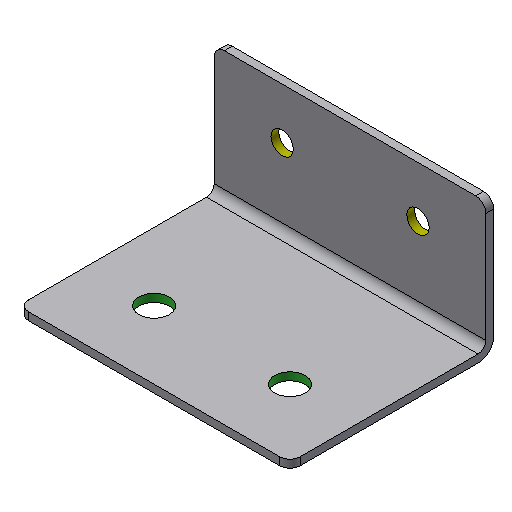
# Autodesk Inventor part: TL20240701-10130CV-002
Saved by Autodesk Inventor 2022.5 (Build 265521000, 521)
## iProperties
Category: JOINT LEG ASSY
Company: 현대 트랜시스(대유)
Created: 2023-04-20
Part Number: TL20240701-10130CV-002
Checked By: 김형민
Engr Approved By: 김시현
User Status: 2 x37
Material: SS400
Description: 0
Document SubType Name: Modeling
Mfg Approved By: 호상태
Designer: 김건휴
Stock Number: 002
Density: 7.85 g/cm^3
Appearance: Painting-RAL7035
Project: SW PJT
DETAIL: Coveryor Assembly
M/C TITLE: CJ 제일제당 협동로봇 포장시스탬 PILOT 장비
PARTS NAME: Bracket
SPECIFICATION: TA20221101-CV200000-015
DocNumber: 221118_Standard_v1
Folder: .\
VDS_Category: 엔지니어링
Detail Description: Processed products
Title: BRACKET
Subject: SW차종 시트조립라인
Author: 김건휴
Revision Number: A
Autodesk Inventor part; units mm, degrees
ref_plane "YZ Plane" through (0, 0, 0) normal (1, 0, 0) x (0, 1, 0)
ref_plane "XZ Plane" through (0, 0, 0) normal (0, 1, 0) x (-1, 0, 0)
ref_plane "XY Plane" through (0, 0, 0) normal (0, 0, 1) x (1, 0, 0)
sketch "스케치9" plane through (0, 0, 0) normal (1, 0, 0) x (0, 1, 0)
  line L0 (2.3, 0) -> (0, 0)
  line L1 (0, 0) -> (0, 60)
  line L2 (0, 60) -> (2.3, 60)
  line L3 (2.3, 60) -> (2.3, 0)
  line L4 (0, 0) -> (40, 0)
  line L5 (40, 0) -> (40, 2.3)
  line L6 (40, 2.3) -> (0, 2.3)
  line L7 (0, 2.3) -> (0, 0)
  point P0 (2.3, 2.3)
  dimension "d40" = 2.3
  dimension "d41" = 2.3
  dimension "d42" = 60
  dimension "d43" = 40
  constraints: 16 end point, 4 parallel, 2 horizontal, 2 perpendicular, 1 coincident
  measures "d40" distance of L4.end L5.end
  measures "d41" distance of L1.end L2.end
  measures "d42" distance of point (0, 0) L1.end
  measures "d43" distance of L0.end L4.end
extrude "돌출4" add sketch "스케치9" along normal blind 80
sketch "스케치10" plane through (0, 2.3, 2.3) normal (0, 0, 1) x (1, 0, 0)
  line L0 (0, 37.7) -> (0, 0) projected
  line L1 (80, 37.7) -> (80, 0) projected
  line L2 (0, -2.3) -> (80, -2.3) projected
  point P0 (20, 22.7)
  point P1 (60, 22.7)
  dimension "d46" = 20
  dimension "d47" = 20
  dimension "d48" = 25
  constraints: 1 horizontal alignment
  measures "d46" distance from line of point (20, 22.7) L0
  measures "d47" distance from line of L1 point (60, 22.7)
  measures "d48" distance from line of point (20, 22.7) L2
hole "구멍3" at (20, 25, 2.3) at (60, 25, 2.3) direction (0, 0, -1) diameter 6.6 end through all clearance for "Slotted Cheese Head Screw ISO 1207" size "M6" standard "ISO"
sketch "스케치11" plane through (0, 2.3, 60) normal (0, 1, 0) x (1, 0, 0)
  line L0 (0, 57.7) -> (0, 0) projected
  line L1 (0, 0) -> (80, 0) projected
  point P0 (0, 60)
  point P1 (20, 20)
  point P2 (60, 20)
  dimension "d56" = 20
  dimension "d57" = 40
  dimension "d58" = 20
  constraints: 1 horizontal alignment
  measures "d56" distance from line of point (20, 20) L0
  measures "d57" distance of point (60, 20) point (20, 20)
  measures "d58" distance from line of L1 point (60, 20)
hole "구멍4" at (20, 2.3, 40) at (60, 2.3, 40) direction (0, -1, 0) diameter 9 end through all clearance for "Socket Head Cap Screw ISO 4762" size "M8" standard "ISO"
fillet "모깎기2" radius 2.3 1 edges at (40, 2.3, 2.3)
fillet "모깎기3" radius 4.6 1 edges at (40, 0, 0)
fillet "모깎기4" radius 3 4 edges at (80, 40, 1.15) (0, 40, 1.15) (80, 1.15, 60) (0, 1.15, 60)
